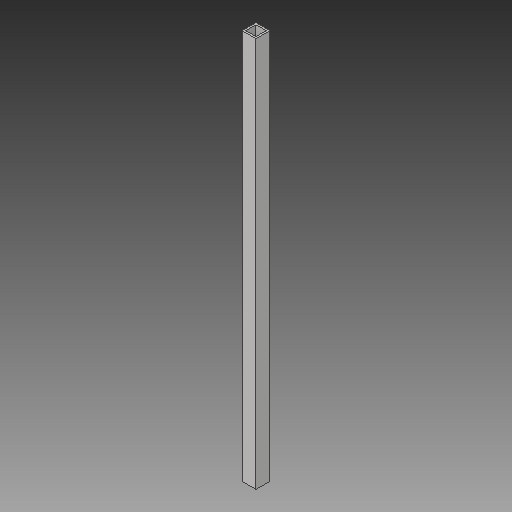
# Autodesk Inventor part: Aluminum channel (Electrical pannel mount)
Saved by Autodesk Inventor 2019 (Build 230136000, 136)
## iProperties
Created: 2019-03-18
Part Number: Aluminum channel (Electrical pannel mount)
Material: Generic
Document SubType Name: Modeling
Designer: josh
Density: 1 g/cm^3
Appearance: Default
Mass: 89.4734 g
Surface Area: 707.87 cm^2
Volume: 89.4734 cm^3
Author: josh
Autodesk Inventor part; units mm, degrees
ref_plane "YZ Plane" through (0, 0, 0) normal (1, 0, 0) x (0, 1, 0)
ref_plane "XZ Plane" through (0, 0, 0) normal (0, 1, 0) x (-1, 0, 0)
ref_plane "XY Plane" through (0, 0, 0) normal (0, 0, 1) x (1, 0, 0)
sketch "Sketch1" plane through (0, 0, 0) normal (0, 1, 0) x (-1, 0, 0)
  line L0 (0, 0) -> (-19.05, 0)
  line L1 (-19.05, 0) -> (-19.05, -19.05)
  line L2 (-19.05, -19.05) -> (0, -19.05)
  line L3 (0, -19.05) -> (0, 0)
  line L4 (-2.54, -2.54) -> (-16.51, -2.54)
  line L5 (-16.51, -2.54) -> (-16.51, -16.51)
  line L6 (-16.51, -16.51) -> (-2.54, -16.51)
  line L7 (-2.54, -16.51) -> (-2.54, -2.54)
  dimension "d0" = 19.05
  dimension "d1" = 19.05
  dimension "d2" = 2.54
  constraints: 16 end point, 4 parallel, 2 perpendicular, 1 horizontal, 3 other
  measures "d0" distance of L2.end L1.end
  measures "d1" distance of L1.end L0.end
  measures "d2" distance between parallel lines of L3 L7
extrude "Extrusion1" add sketch "Sketch1" along normal blind 533.4
body "Solid1"
